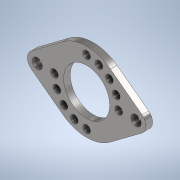
# Autodesk Inventor part: Pancake Mount Plate
Saved by Autodesk Inventor 2021 (Build 250183000, 183)
## iProperties
Created: 2021-02-26
Part Number: Pancake Mount Plate
Material: Steel, Galvanized
Document SubType Name: Modeling
Designer: aidan
Density: 7.85 g/cm^3
Appearance: Galvanized
Author: aidan
Autodesk Inventor part; units mm, degrees
ref_plane "YZ Plane" through (0, 0, 0) normal (1, 0, 0) x (0, 1, 0)
ref_plane "XZ Plane" through (0, 0, 0) normal (0, 1, 0) x (-1, 0, 0)
ref_plane "XY Plane" through (0, 0, 0) normal (0, 0, 1) x (1, 0, 0)
sketch "Sketch1" plane through (0, 0, 0) normal (0, 0, 1) x (1, 0, 0)
  line L0 (-11.4198, 15.2476) -> (-26.6751, 3.8221)
  line L1 (-26.6751, -3.8221) -> (-11.4198, -15.2476)
  line L2 (11.4198, 15.2476) -> (26.6751, 3.8221)
  line L3 (26.6751, -3.8221) -> (11.4198, -15.2476)
  line L4 (-31.7782, 0) -> (31.7782, 0) construction
  arc A0 (-26.6751, 3.8221) -> (-26.6751, -3.8221) centre (-23.8125, 0) ccw
  arc A1 (26.6751, -3.8221) -> (26.6751, 3.8221) centre (23.8125, 0) ccw
  arc A2 (-11.4198, -15.2476) -> (11.4198, -15.2476) centre (0, 0) ccw
  arc A3 (11.4198, 15.2476) -> (-11.4198, 15.2476) centre (0, 0) ccw
  dimension "d1" = 4.7752
  dimension "d2" = 47.625
  constraints: 10 end point, 8 point on circle, 8 tangent, 4 centre point, 4 point on line, 1 coincident, 1 equal length, 1 equal radius, 1 horizontal, 1 midpoint
  measures "d1" radius of A0
  measures "d2" distance of A1.centre A0.centre
extrude "Extrusion1" add sketch "Sketch1" along normal blind 3.175
sketch "Sketch2" plane through (0, 0, 3.175) normal (0, 0, 1) x (1, 0, 0)
  arc A0 (-26.6751, 3.8221) -> (-26.6751, -3.8221) centre (-23.8125, 0) ccw projected
  arc A1 (26.6751, -3.8221) -> (26.6751, 3.8221) centre (23.8125, 0) ccw projected
  circle A2 centre (-23.8125, 0) radius 2.4892
  circle A3 centre (23.8125, 0) radius 2.4892
  circle A4 centre (0, 0) radius 11.1125
  dimension "d5" = 22.225
  dimension "d6" = 4.9784
  constraints: 3 centre point, 3 coincident, 1 equal radius
  measures "d5" diameter of A4
  measures "d6" diameter of A2
extrude "Extrusion2" cut sketch "Sketch2" against normal blind 3.175
sketch "Sketch3" plane through (0, 0, 3.175) normal (0, 0, 1) x (1, 0, 0)
  arc A0 (11.4198, 15.2476) -> (-11.4198, 15.2476) centre (0, 0) ccw projected
  line L0 (0, 19.05) -> (0, -19.6536) construction
  circle A1 centre (0, 15.494) radius 1.8288
  circle A2 centre (0, -15.494) radius 1.8288
  dimension "d9" = 30.988
  dimension "d10" = 15.494
  dimension "d11" = 3.6576
  constraints: 3 point on line, 2 centre point, 2 end point, 1 equal radius, 1 point on circle, 1 vertical
  measures "d9" distance of A2.centre A1.centre
  measures "d10" distance of point (0, 0) A1.centre
  measures "d11" diameter of A1
extrude "Extrusion3" cut sketch "Sketch3" against normal blind 3.175
pattern_circular "Circular Pattern1" count 5 over 90 about axis through (0, 0, 3.175) along (0, 0, -1) of "Extrusion3"
body "Solid1"
